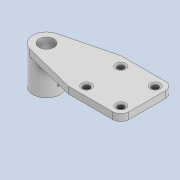
# Autodesk Inventor part: WM 720p USB Webcam Endefector Mount
Saved by Autodesk Inventor 2022 (Build 260153000, 153)
## iProperties
Created: 2021-10-12
Part Number: WM 720p USB Webcam Endefector Mount
Material: Generic
Document SubType Name: Modeling
Designer: Coy
Density: 1 g/cm^3
Appearance: Default
Author: Coy
Autodesk Inventor part; units mm, degrees
ref_plane "YZ Plane" through (0, 0, 0) normal (1, 0, 0) x (0, 1, 0)
ref_plane "XZ Plane" through (0, 0, 0) normal (0, 1, 0) x (-1, 0, 0)
ref_plane "XY Plane" through (0, 0, 0) normal (0, 0, 1) x (1, 0, 0)
sketch "Sketch1" plane through (0, 0, 0) normal (0, 1, 0) x (-1, 0, 0)
  circle A0 centre (0, 0) radius 3.25
  circle A1 centre (0, 0) radius 6
  dimension "d0" = 6.5
  dimension "d1" = 12
  constraints: 2 centre point, 2 coincident
  measures "d0" diameter of A0
  measures "d1" diameter of A1
extrude "Extrusion1" add sketch "Sketch1" along normal blind 13.5
sketch "Sketch2" plane through (0, 13.5, 0) normal (0, 1, 0) x (1, 0, 0)
  line L0 (0, 0) -> (25, 0) construction
  line L1 (25, 7.5) -> (40, 7.5) construction
  line L2 (40, 7.5) -> (40, -7.5) construction
  line L3 (40, -7.5) -> (25, -7.5) construction
  line L4 (25, -7.5) -> (25, 7.5) construction
  circle A0 centre (25, 7.5) radius 1.4
  circle A1 centre (40, 7.5) radius 1.4
  circle A2 centre (40, -7.5) radius 1.4
  circle A3 centre (25, -7.5) radius 1.4
  circle A4 centre (0, 0) radius 6.3 construction
  line L5 (40.5, 11.5) -> (21, 11.5)
  line L6 (21, -11.5) -> (40.5, -11.5)
  line L7 (44, -8) -> (44, 8)
  line L8 (21, 11.5) -> (-1.4711, 5.8169)
  line L9 (21, -11.5) -> (-1.4711, -5.8169)
  circle A5 centre (0, 0) radius 6 projected
  circle A6 centre (0, 0) radius 3.25 projected
  arc A7 (44, 8) -> (40.5, 11.5) centre (40.5, 8) ccw
  arc A8 (40.5, -11.5) -> (44, -8) centre (40.5, -8) ccw
  dimension "d4" = 25
  dimension "d5" = 15
  dimension "d6" = 15
  dimension "d7" = 7.5
  dimension "d8" = 2.8
  dimension "d9" = 2.8
  dimension "d10" = 2.8
  dimension "d11" = 2.8
  dimension "d12" = 12.6
  dimension "d13" = 4
  dimension "d14" = 3.5
  constraints: 20 end point, 7 centre point, 6 point on circle, 6 tangent, 5 coincident, 3 parallel, 2 horizontal, 2 perpendicular, 1 equal radius, 1 other
  measures "d4" distance of L0.start L0.end
  measures "d5" distance of L2.end L3.end
  measures "d6" distance of L1.end L2.end
  measures "d7" distance between parallel lines of L0 L1
  measures "d8" diameter of A0
  measures "d9" diameter of A1
  measures "d10" diameter of A2
  measures "d11" diameter of A3
  measures "d12" diameter of A4
  measures "d13" distance between parallel lines of L1 L5
  measures "d14" radius of A7
extrude "Extrusion2" add sketch "Sketch2" along normal blind 3
fillet "Fillet1" radius 0.8 4 edges at (23.6, 16.5, 7.5) (23.6, 16.5, -7.5) (38.6, 16.5, -7.5) (38.6, 16.5, 7.5)
sketch "Sketch3" plane through (0, 13.5, 0) normal (0, -1, 0) x (1, 0, 0)
  circle A0 centre (0, 0) radius 6 projected
  line L0 (5.9161, 1) -> (16, 1)
  line L1 (5.9161, -1) -> (16, -1)
  line L2 (16, 1) -> (16, -1)
  dimension "d18" = 1
  dimension "d19" = 1
  dimension "d20" = 10
  constraints: 6 end point, 2 horizontal, 2 point on circle, 1 perpendicular
  measures "d18" distance from line of point (0, 0) L0
  measures "d19" distance from line of point (0, 0) L1
  measures "d20" distance edge to line of A0 L2
extrude "Extrusion3" add sketch "Sketch3" along normal blind 10 contours A0 L0 L2 L1
chamfer "Chamfer1" distance 10 angle 45 1 edges at (16, 3.5, 0)
equation "\"d7\" = 0.5 * d6"
equation "\"d9\" = d8"
equation "\"d10\" = d8"
equation "\"d11\" = d8"
body "Solid1"
